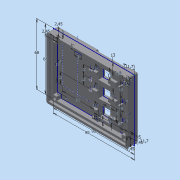
# Autodesk Inventor part: TopV2
Saved by Autodesk Inventor 2015 (Build 190159000, 159)
## iProperties
Created: 2014-12-30
Part Number: TopV2
Material: Generic
Document SubType Name: Modeling
Designer: Openlab
Density: 1 g/cm^3
Appearance: Default
Author: Openlab
Autodesk Inventor part; units mm, degrees
ref_plane "YZ Plane" through (0, 0, 0) normal (1, 0, 0) x (0, 1, 0)
ref_plane "XZ Plane" through (0, 0, 0) normal (0, 1, 0) x (-1, 0, 0)
ref_plane "XY Plane" through (0, 0, 0) normal (0, 0, 1) x (1, 0, 0)
sketch "Sketch1" plane through (0, 0, 0) normal (0, 1, 0) x (-1, 0, 0)
  line L0 (5, -5) -> (5, -63)
  line L1 (5, -63) -> (85, -63)
  line L2 (85, -63) -> (85, -5)
  line L3 (34.7, -6.5) -> (21.7, -6.5)
  line L4 (21.7, -6.5) -> (21.7, -19.5)
  line L5 (21.7, -19.5) -> (34.7, -19.5)
  line L6 (21.7, -42.5) -> (21.7, -55.5)
  line L7 (21.7, -55.5) -> (34.7, -55.5)
  line L8 (34.7, -42.5) -> (21.7, -42.5)
  line L9 (85, -63) -> (81, -63)
  line L10 (81, -63) -> (81, -59)
  line L11 (81, -59) -> (85, -59)
  line L12 (85, -59) -> (85, -63)
  line L13 (5, -5) -> (9, -5)
  line L14 (9, -5) -> (9, -9)
  line L15 (9, -9) -> (5, -9)
  line L16 (5, -9) -> (5, -5)
  line L17 (5, -63) -> (9, -63)
  line L18 (9, -63) -> (9, -59)
  line L19 (9, -59) -> (5, -59)
  line L20 (5, -59) -> (5, -63)
  line L21 (85, -5) -> (51.4243, -5)
  line L22 (39.7, -59) -> (11.7, -59)
  line L23 (34.7, -50.25) -> (39.7, -50.25)
  line L24 (39.7, -47.75) -> (34.7, -47.75)
  line L25 (39.7, -32.25) -> (34.7, -32.25)
  line L26 (39.7, -29.75) -> (34.7, -29.75)
  line L27 (34.7, -14.25) -> (39.7, -14.25)
  line L28 (34.7, -11.75) -> (39.7, -11.75)
  line L29 (11.7, -51.25) -> (21.7, -51.25)
  line L30 (11.7, -46.75) -> (21.7, -46.75)
  line L31 (11.7, -33.25) -> (21.7, -33.25)
  line L32 (11.7, -28.75) -> (21.7, -28.75)
  line L33 (11.7, -15.25) -> (21.7, -15.25)
  line L34 (11.7, -10.75) -> (21.7, -10.75)
  line L35 (41.4, -5) -> (41.4, -59)
  line L36 (85, -5) -> (44.4, -5)
  line L37 (41.4, -5) -> (39.7, -5)
  line L38 (38.4, -63) -> (38.4, -61)
  line L39 (41.4, -5) -> (44.4, -5)
  line L40 (10, -5) -> (10, -63)
  line L41 (41.4, -59) -> (44.4, -59)
  line L42 (44.4, -63) -> (44.4, -61)
  line L43 (44.4, -59) -> (44.4, -5)
  line L44 (44.4, -61) -> (38.4, -61)
  line L45 (38.3911, -13) -> (10.1743, -13) construction
  line L46 (34.7, -6.5) -> (34.7, -19.5)
  line L47 (40.371, -31) -> (7.5475, -31) construction
  line L48 (9.897, -49) -> (40.0785, -49) construction
  line L49 (39.7, -5) -> (39.7, -59)
  line L50 (34.7, -42.5) -> (34.7, -55.5)
  line L51 (34.7, -24.5) -> (21.7, -24.5)
  line L52 (21.7, -24.5) -> (21.7, -37.5)
  line L53 (21.7, -37.5) -> (34.7, -37.5)
  line L54 (34.7, -37.5) -> (34.7, -24.5)
  line L55 (81, -5) -> (81, -9)
  line L56 (81, -9) -> (85, -9)
  line L57 (13.2, -46.75) -> (13.2, -51.25)
  line L58 (13.2, -28.75) -> (13.2, -33.25)
  line L59 (13.2, -10.75) -> (13.2, -15.25)
  line L60 (39.7, -5) -> (9, -5)
  line L61 (11.7, 0) -> (11.7, -68)
  line L62 (45, -5) -> (45, -50) construction
  line L63 (80, -50) -> (80, -5) construction
  line L64 (80, -5) -> (45, -5)
  line L65 (45, -50) -> (80, -50) construction
  line L66 (62.5, 6.7089) -> (62.5, -52.768) construction
  line L67 (66.5, -10) -> (58.5, -10)
  line L68 (58.5, -10) -> (58.5, -5)
  line L69 (66.5, -5) -> (66.5, -10)
  line L70 (87.55, -2.45) -> (2.45, -2.45)
  line L71 (2.45, -2.45) -> (2.45, -65.55)
  line L72 (2.45, -65.55) -> (87.55, -65.55)
  line L73 (87.55, -65.55) -> (87.55, -2.45)
  line L74 (90, -68) -> (0, -68)
  line L75 (0, -68) -> (0, 0)
  line L76 (0, 0) -> (90, 0)
  line L77 (90, 0) -> (90, -68)
  point P0 (49, -38)
  point P1 (49, -28)
  point P2 (49, -18)
  point P3 (11.7, -5)
  point P4 (11.7, -63)
  dimension "d4" = 13
  dimension "d8" = 4
  dimension "d9" = 4
  dimension "d11" = 4
  dimension "d24" = 2.5
  dimension "d27" = 4.5
  dimension "d28" = 4.5
  dimension "d29" = 4.5
  dimension "d34" = 2
  dimension "d40" = 3
  dimension "d41" = 6
  dimension "d43" = 13
  dimension "d45" = 18
  dimension "d46" = 18
  dimension "d47" = 13
  dimension "d48" = 5
  dimension "d49" = 1.7
  dimension "d51" = 13
  dimension "d52" = 2.5
  dimension "d53" = 2.5
  dimension "d65" = 8.5
  dimension "d116" = 35
  dimension "d117" = 45
  dimension "d124" = 8
  dimension "d125" = 5
  dimension "d141" = 12
  dimension "d142" = 10
  dimension "d143" = 10
  dimension "d154" = 1
  dimension "d156" = 4
  dimension "d165" = 3.5
  dimension "d171" = 4
  dimension "d173" = 5
  dimension "d176" = 10
  dimension "d177" = 1.7
  dimension "d196" = 5
  dimension "d197" = 5
  dimension "d198" = 5
  dimension "d199" = 5
  dimension "d200" = 13
  dimension "d201" = 2.45
  dimension "d202" = 2.45
  dimension "d203" = 2.45
  dimension "d204" = 2.45
  dimension "d205" = 68
  dimension "d206" = 90
  dimension "d218" = 11.7
  constraints: 154 end point, 39 point on line, 23 parallel, 23 perpendicular, 19 horizontal, 12 collinear, 5 vertical, 2 vertical alignment, 1 coincident, 23 other
  measures "d4" distance of L7.end L8.start
  measures "d8" distance of L10.end L11.end
  measures "d9" distance of L9.end L10.end
  measures "d11" distance of L13.end L14.end
  measures "d24" distance between parallel lines of L26 L25
  measures "d27" distance between parallel lines of L34 L33
  measures "d28" distance between parallel lines of L32 L31
  measures "d29" distance between parallel lines of L29 L30
  measures "d34" distance of L38.start L38.end
  measures "d40" distance of L35.end L41.end
  measures "d41" distance of L42.end L38.end
  measures "d43" distance between parallel lines of L5 L3
  measures "d45" distance between parallel lines of L47 L45
  measures "d46" distance between parallel lines of L48 L47
  measures "d47" distance between parallel lines of L6 L50
  measures "d48" distance between parallel lines of L50 L49
  measures "d49" distance between parallel lines of L49 L35
  measures "d51" distance between parallel lines of L53 L51
  measures "d52" distance between parallel lines of L27 L28
  measures "d53" distance between parallel lines of L23 L24
  measures "d65" distance between parallel lines of L4 L59
  measures "d116" distance of L63.start L62.end
  measures "d117" distance of L63.end L63.start
  measures "d124" distance of L67.start L67.end
  measures "d125" distance of L69.start L67.start
  measures "d141" distance from line of L65 point (49, -38)
  measures "d142" distance of point (49, -38) point (49, -28)
  measures "d143" distance of point (49, -28) point (49, -18)
  measures "d154" distance between parallel lines of L40 L14
  measures "d156" distance of L14.end L15.end
  measures "d165" distance between parallel lines of L7 L22
  measures "d171" distance from line of L62 point (49, -18)
  measures "d173" distance between parallel lines of L2 L63
  measures "d196" distance between parallel lines of L77 L2
  measures "d197" distance between parallel lines of L76 L21
  measures "d198" distance between parallel lines of L75 L0
  measures "d199" distance between parallel lines of L74 L1
  measures "d200" distance between parallel lines of L76 L45
  measures "d201" distance between parallel lines of L77 L73
  measures "d202" distance between parallel lines of L76 L70
  measures "d203" distance between parallel lines of L75 L71
  measures "d204" distance between parallel lines of L74 L72
  measures "d205" distance of L76.end L74.start
  measures "d206" distance of L74.start L74.end
sketch "Sketch5" plane through (0, 0, 0) normal (0, 1, 0) x (-1, 0, 0)
  line L0 (0, 0) -> (90, 0)
  line L1 (90, 0) -> (90, -68)
  line L2 (90, -68) -> (0, -68)
  line L3 (0, -68) -> (0, 0)
  line L4 (11.7, -68) -> (11.7, 0)
  line L5 (44.7, -68) -> (44.7, 0)
  dimension "d219" = 90
  dimension "d220" = 68
  dimension "d221" = 11.7
  dimension "d222" = 33
  constraints: 12 end point, 4 point on line, 3 perpendicular, 2 parallel, 1 horizontal
  measures "d219" distance of L1.end L2.end
  measures "d220" distance of L0.end L1.end
  measures "d221" distance between parallel lines of L3 L4
  measures "d222" distance between parallel lines of L4 L5
extrude "Extrusion28" add sketch "Sketch5" along normal blind 5 contours L0 L4 L2 L3 | L0 L1 L2 L5
extrude "Extrusion29" add sketch "Sketch5" along normal blind 3.5 contours L0 L5 L2 L4
extrude "Extrusion30" add sketch "Sketch1" against normal blind 7.5 contours L70 L71 L72 L61 L74 L75 L76 | L61 L76 L77 L74 L72 L73 L70
extrude "Extrusion31" add sketch "Sketch1" against normal blind 5 contours L13 L14 L15 L0 | L0 L1 L61 L72 L71 L70 L60 L13 | L19 L18 L1 L0 | L61 L70 L73 L72 L1 L2 L21 L36 L39 L37 L60 | L60 L49 L28 L46 L3 L4 L34 L61 | L61 L29 L6 L7 L50 L23 L49 L22 | L33 L4 L5 L46 L27 L49 L26 L54 L51 L52 L32 L61 | L10 L11 L2 L1 | L61 L31 L52 L53 L54 L25 L49 L24 L50 L8 L6 L30 | L56 L55 L21 L2
extrude "Extrusion32" add sketch "Sketch1" against normal blind 2.5 contours L15 L14 L60 L40 L1 L18 L19 L0 | L38 L44 L42 L1 | L39 L43 L41 L35
extrude "Extrusion33" add sketch "Sketch1" against normal blind 7.5 contours L49 L27 L46 L28 | L34 L4 L33 L59 | L23 L50 L24 L49 | L57 L30 L6 L29 | L49 L25 L54 L26 | L32 L52 L31 L58
extrude "Extrusion34" cut sketch "Sketch1" along normal through all contours L46 L5 L4 L3 | L50 L7 L6 L8 | L54 L53 L52 L51
sketch "Sketch6" plane through (0, 5, 0) normal (0, 1, 0) x (1, 0, 0)
  line L0 (-44.7, 68) -> (-90, 68) projected
  line L1 (-90, 68) -> (-90, 0) projected
  point P0 (0, 0)
  point P1 (-6, 6)
  point P2 (-6, 62)
  point P3 (-84, 62)
  point P4 (-84, 6)
  dimension "d237" = 6
  dimension "d238" = 6
  dimension "d239" = 6
  dimension "d240" = 6
  constraints: 2 horizontal alignment, 2 vertical alignment
  measures "d237" horizontal distance of point (0, 0) point (-6, 6)
  measures "d238" horizontal distance of point (0, 0) point (-6, 6)
  measures "d239" distance from line of L0 point (-84, 62)
  measures "d240" distance from line of L1 point (-84, 62)
hole "Hole4" at (-6, 5, -6) at (-6, 5, -62) at (-84, 5, -62) at (-84, 5, -6) direction (0, -1, 0) diameter 4 end through all counterbore diameter 6.5 counterbore depth 3
fillet "Fillet5" radius 2 24 edges at (-67.35, 5, 0) (-90, 5, -34) (-67.35, 5, -68) (-28.2, 3.5, -68) (-5.85, 5, -68) (0, 5, -34) (-28.2, 3.5, 0) (-5.85, 5, 0) (-28.2, 3.5, -6.5) (-34.7, 3.5, -13) (-28.2, 3.5, -19.5) (-21.7, 3.5, -13) (-28.2, 3.5, -24.5) (-34.7, 3.5, -31) (-21.7, 3.5, -31) (-28.2, 3.5, -37.5) (-28.2, 3.5, -42.5) (-34.7, 3.5, -49) (-28.2, 3.5, -55.5) (-21.7, 3.5, -49) (0, -1.25, 0) (0, -1.25, -68) (-90, -1.25, -68) (-90, -1.25, 0)
hole "Hole5" at (-49, 0, -38) at (-49, 0, -28) at (-49, 0, -18) direction (0, 1, 0) diameter 5.5 end through all
body "Solid4"
